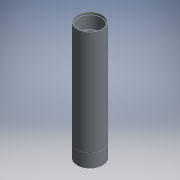
# Autodesk Inventor part: SLZ_63_Schubstange#_274.5_1001
Saved by Autodesk Inventor 2017.3 (Build 213256000, 256)
## iProperties
Part Number: SLZ_63_Schubstange#_274.5_1001
Material: Generic
Catalog Web Link: www.cadenas.de
Description: Schubstange SLZ63-Control-Tec
Vendor: ROSEKRIEGER
Document SubType Name: Modeling
Designer: partserver
Manufacturer: ROSEKRIEGER
Mass: 77.3426 g
Surface Area: 427.24 cm^2
Volume: 77.3426 cm^3
Density: 1 g/cm^3
Appearance: PSOLRGB-157-164-172
Category: PARTsolutions
Company: ROSEKRIEGER
Title: SLZ_63_Schubstange#_274.5_1001
Author: Cadenas PARTsolutions
Comments: Control-Tec
PSOL_IDENT_0: {$CADENAS_DATA\23d-libs\rose_krieger\linearkomponenten\pool_lineartechnik\_hubsaeule_zyliinder\elekt
PSOL_IDENT_1: rozylinder\elekzyl_slz63\parts\slz63_plfl_schubstange.prj},213 {VTYP=3D},{NB=SLZ_63_Schubstange#_274
PSOL_IDENT_2: .5_1001},{LINA=SLZ_63_Schubstange#_274.5_1001},{NN=Schubstange SLZ63},{DATE=02.12.2020 11:16:24},{GE
PSOL_IDENT_3: OMDATE=01.03.2017 14:14:13},{VERSION=},{LINEID=1700},{WBVAR=},{WBNUMERIC=}  {NB=SLZ_63_Schubstange#_
PSOL_IDENT_4: 274.5_1001},{LINA=SLZ_63_Schubstange#_274.5_1001},{KT=DUMMY},{IDNR=},{CODE=TQ3},{ARTIKEL=Elektrozyli
PSOL_IDENT_5: nder },{TYPE=SLZ 63 Tr P PL},{BEST=SLZ_63_Schubstange},{VARIANTE=PL},{SPINDEL=Tr 28x10},{SPINDELCODE=
PSOL_IDENT_6: 1.000},{SCHUTZARTVIS=IP54},{SCHUTZART=1},{HUB1=0,[0:100]},{HUB2=100},{L2=184},{HINWEINBAUX=Hub + 274
PSOL_IDENT_7: ,5 mm},{DUMMYDURCH=10.000},{DUMMYLAENG=20.000},{HILFEHUB=105},{LAENDOPPROFIL=184.500},{RF=1.000},{GR
PSOL_IDENT_8: UNDKOE=274.500},{A=100},{B=80},{C=100},{D=125},{E=238},{F=40},{G=M16x1.5},{H=104},{K=125},{L=105},{M=
PSOL_IDENT_9: 48},{N=56.5},{O=86},{P=18.5},{PPATH=sbl_lz70p_plfl.prj}
NB: SLZ_63_Schubstange#_274.5_1001
NN: Schubstange SLZ63
NT: Control-Tec
NBSYN: $BEST.#_$GRUNDKOE._$HUB2.$SCHUTZART.
LINA: SLZ_63_Schubstange#_274.5_1001
CATALOG: RK Rose+Krieger
CODE: TQ3
ARTIKEL: Elektrozylinder
BEST: SLZ_63_Schubstange
VARIANTE: PL
SPINDEL: Tr 28x10
SPINDELCODE: 1
SCHUTZARTVIS: IP54
SCHUTZART: 1
HUB1: 0,[0:100]
L2: 184
HINWEINBAUX: Hub + 274,5 mm
DUMMYDURCH: 10
DUMMYLAENG: 20
HILFEHUB: 105
LAENDOPPROFIL: 184.5
RF: 1
GRUNDKOE: 274.5
A: 100
B: 80
C: 100
D: 125
E: 238
F: 40
G: M16x1.5
H: 104
K: 125
L: 105
M: 48
N: 56.5
O: 86
P: 18.5
SUPPLIER: ROSEKRIEGER
ARTICLENO: SLZ_63_Schubstange#_274.5_1001
BOMINFO: SLZ_63_Schubstange#_274.5_1001
CREATOR: CADENAS GmbH
Autodesk Inventor part; units mm, degrees
sketch "Sketch_1" plane through (0, 0, 0) normal (1, 0, 0) x (0, 0, -1)
  line L0 (0, 0) -> (-184, 0)
  line L1 (-184, 19.7) -> (-184, 17.75)
  line L2 (-184, 17.75) -> (-183.5, 17.25)
  line L3 (-183.5, 17.25) -> (-165, 17.25)
  line L4 (-165, 17.25) -> (-164.2489, 16)
  line L5 (-164.2489, 16) -> (-22.7511, 16)
  line L6 (-22.7511, 16) -> (-22, 17.25)
  line L7 (-22, 17.25) -> (-3, 17.25)
  line L8 (-3, 17.25) -> (-3, 18.5)
  line L9 (-3, 18.5) -> (0, 18.5)
  line L10 (0, 18.5) -> (0, 20)
  line L11 (0, 20) -> (-162.7709, 20)
  arc A0 (-163.2291, 20) -> (-162.7709, 20) centre (-163, 20.1) ccw
  line L12 (-163.2291, 20) -> (-183.7, 20)
  line L13 (-183.7, 20) -> (-184, 19.7)
  constraints: 28 end point, 2 point on circle, 1 centre point
revolve "Revolution1" add sketch "Sketch_1" angle 360 about axis through (0, 0, 0) along (0, 0, -1)
ref_plane "ABDECKKAPPE_XY" through (0, 0, 158) normal (0, 0, 1) x (1, 0, 0)
ref_plane "ABDECKKAPPE_YZ" through (0, 0, 158) normal (1, 0, 0) x (0, 1, 0)
ref_plane "ABDECKKAPPE_ZX" through (0, 0, 158) normal (0, 1, 0) x (0, 0, 1)
ref_plane "SCHUBSTANGE_XY" through (0, 0, 184) normal (0, 0, -1) x (1, 0, 0)
ref_plane "SCHUBSTANGE_YZ" through (0, 0, 184) normal (1, 0, 0) x (0, -1, 0)
ref_plane "SCHUBSTANGE_ZX" through (0, 0, 184) normal (0, -1, 0) x (0, 0, -1)
body "Solid1"
